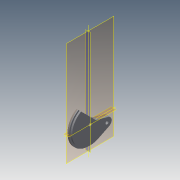
# Autodesk Inventor part: HbIndexInputLink01
Saved by Autodesk Inventor 2015 SP1 (Build 190203100, 203)
## iProperties
Created: 2015-02-15
Part Number: HbIndexInputLink01
Material: 一般
Document SubType Name: Modeling
Designer: Yamaura
Density: 1 g/cm^3
Appearance: 既定
Author: Yamaura
Autodesk Inventor part; units mm, degrees
sketch "スケッチ1" plane through (0, 0, 0) normal (1, 0, 0) x (0, 1, 0)
  circle A0 centre (0, 0) radius 12
  circle A1 centre (11.086554, -4.592201) radius 1
  line L0 (11.999999, 0.003871) -> (0, 0)
  circle A2 centre (0, 36.4) radius 3.05
  line L1 (0, -24.29622) -> (0, 61.777317)
  line L2 (-17.517311, 0) -> (21.103865, 0)
  line L3 (0, 0) -> (11.086554, 4.592201)
  line L4 (0, 0) -> (12, 0) construction
  line L5 (7.00243, 39.302753) -> (11.086554, 4.592201)
  circle A3 centre (11.086554, 4.592201) radius 4.5
  line L6 (1.095705, 28.899371) -> (0, 36.4)
  circle A4 centre (0, 0) radius 1
  line L7 (0, 0) -> (11.086554, -4.592201)
  line L8 (1.095705, 28.899371) -> (11.086554, -4.592201)
  line L9 (0, 36.4) -> (0.007491, 49.481097)
  line L10 (0, 36.4) -> (-0.004295, 28.900001)
  line L11 (-0.004295, 28.900001) -> (1.095705, 28.899371)
  line L12 (0, 36.4) -> (-11.643954, 33.459716)
  line L13 (7.271744, 38.236231) -> (0, 36.4)
  line L14 (7.00243, 39.302753) -> (7.271744, 38.236231)
  line L15 (0, 36.4) -> (7.00243, 39.302753)
  dimension "d0" = 24
  dimension "d1" = 2
  dimension "d2" = 6.1
  dimension "d3" = 36.4
  dimension "d5" = 12
  dimension "d7" = 12
  dimension "d11" = 34.95
  dimension "d13" = 9
  dimension "d31" = 2
  dimension "d37" = 34.95
  dimension "d54" = 7.5
  dimension "d55" = 1.1
  dimension "d57" = 7.5
  dimension "d61" = 1.1
  dimension "d62" = 45
  dimension "d66" = 104.205
  dimension "d68" = 22.5
  constraints: 28 end point, 4 centre point, 3 coincident, 2 collinear, 2 perpendicular, 1 equal length, 1 horizontal, 1 point on line, 2 other
  measures "d1" diameter of A1
  measures "d2" diameter of A2
  measures "d3" distance from line of L6.end L2
  measures "d5" distance of L7.end point (0, 0)
  measures "d7" distance of L0.end L3.end
  measures "d11" distance of L5.start L3.end
  measures "d13" diameter of A3
  measures "d31" diameter of A4
  measures "d37" distance of L7.end L6.start
  measures "d54" distance of L6.end L10.end
  measures "d55" distance of L10.end L6.start
  measures "d57" distance of L13.start L6.end
  measures "d61" distance of L5.start L13.start
  measures "d62" angle of L3 L7
  measures "d66" angle of L9 L12
  measures "d68" angle of L7 L4
sketch "スケッチ2" plane through (0, 0, 0) normal (1, 0, 0) x (0, 1, 0)
  circle A0 centre (0, 0) radius 12
  circle A1 centre (11.086554, -4.592201) radius 3
  line L0 (12.405919, -7.286506) -> (5.27746, -10.777217)
  line L1 (-17.517311, 0) -> (21.103865, 0)
  line L2 (13.924647, -3.619972) -> (11.352371, 3.888916)
  circle A2 centre (11.086554, -4.592201) radius 1
  line L3 (0, 0) -> (11.086554, -4.592201)
  dimension "d17" = 24
  dimension "d18" = 6
  dimension "d19" = 12
  dimension "d29" = 2
  dimension "d38" = 22.5
  constraints: 6 end point, 4 point on circle, 4 tangent, 3 centre point, 1 coincident, 1 concentric
  measures "d17" diameter of A0
  measures "d18" diameter of A1
  measures "d19" distance of L3.start A1.centre
  measures "d29" diameter of A2
  measures "d38" angle of L3 L1
extrude "押し出し2" add sketch "スケッチ2" along normal mid plane 3
sketch "スケッチ3" plane through (0, 0, 0) normal (1, 0, 0) x (0, 1, 0)
  circle A0 centre (11.086554, -4.592201) radius 1
  circle A1 centre (0, 0) radius 1
  line L0 (0, 61.777317) -> (0, -24.29622)
  line L1 (0, 0) -> (11.086554, -4.592201)
  dimension "d24" = 2
  dimension "d25" = 2
  dimension "d39" = 12
  dimension "d40" = 67.5
  constraints: 2 centre point, 2 end point, 1 coincident
  measures "d24" diameter of A0
  measures "d25" diameter of A1
  measures "d39" distance of L1.start L1.end
  measures "d40" angle of L1 L0
extrude "押し出し3" cut sketch "スケッチ3" along normal mid plane 3
sketch "スケッチ4" plane through (0, 0, 0) normal (1, 0, 0) x (0, 1, 0)
  circle A0 centre (0, 0) radius 1
  arc A1 (12.75, 0) -> (0, -12.75) centre (0, 0) ccw
  line L0 (0, -12.75) -> (0, -1)
  line L1 (1, 0) -> (12.75, 0)
  line L2 (0, 0) -> (14.050204, 0)
  line L3 (0, 0) -> (0, -18.196867)
  arc A2 (1, 0) -> (0, -1) centre (0, 0) ccw
  dimension "d41" = 25.5
  constraints: 8 end point, 6 point on circle, 4 point on line, 2 centre point, 2 coincident, 2 vertical, 1 horizontal, 1 perpendicular
  measures "d41" diameter of A1
extrude "押し出し4" add sketch "スケッチ4" along normal mid plane 1 contours A0 L0 A1 L1
sketch "スケッチ5" plane through (0, 0, 0) normal (1, 0, 0) x (0, 1, 0)
  line L0 (0, 0) -> (-8.485281, 8.485281)
  line L1 (0, 0) -> (12, 0) construction
  circle A0 centre (11.086554, -4.592201) radius 1
  circle A1 centre (0, 0) radius 1
  arc A2 (11.352371, 3.888916) -> (5.27746, -10.777217) centre (0, 0) ccw
  line L2 (5.27746, -10.777217) -> (12.405919, -7.286506)
  arc A3 (12.405919, -7.286506) -> (13.924647, -3.619972) centre (11.086554, -4.592201) ccw
  line L3 (13.924647, -3.619972) -> (11.352371, 3.888916)
  arc A4 (13.924647, -3.619972) -> (11.900646, -1.704771) centre (11.086554, -4.592201) ccw
  line L4 (-7.185935, 11.428576) -> (3.609889, 0.632751)
  arc A5 (12.771418, 4.37503) -> (-7.185935, 11.428576) centre (0, 0) ccw
  line L5 (12.771418, 4.37503) -> (15.169896, -2.626513)
  line L6 (15.169896, -2.626513) -> (13.414811, -2.131679)
  line L7 (11.900646, -1.704771) -> (3.609889, 0.632751)
  line L8 (13.414811, -2.131679) -> (13.924647, -3.619972)
  point P0 (-6.094518, 10.337159)
  dimension "d44" = 135
  dimension "d46" = 12
  dimension "d47" = 3
  dimension "d50" = 1.5
  constraints: 15 end point, 5 point on circle, 4 tangent, 3 point on line, 2 centre point, 1 coincident, 1 collinear, 1 equal length, 1 horizontal
  measures "d44" angle of L1 L0
  measures "d46" distance of L0.start L0.end
  measures "d47" distance between parallel lines of L0 L4
  measures "d50" radial gap between concentric circles of A2 A5
extrude "押し出し5" cut sketch "スケッチ5" along normal through all both and the other way through all contours L4 A5 L5 L6 L3 A2 | A2 L3 A4 L7 L4
offset faces "サイズ1" outward 0.25 faces at (0.166667, -9.020805, -9.010414)
